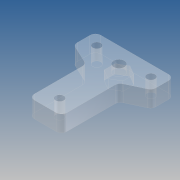
# Autodesk Inventor part: adapterplatte
Saved by Autodesk Inventor 2011 (Build 150239000, 239)
## iProperties
Created: 2014-03-14
Part Number: adapterplatte
Document SubType Name: Modeling
Designer: Kretschmer
Density: 1 g/cm^3
Author: Kretschmer
Autodesk Inventor part; units mm, degrees
ref_plane "YZ Plane" through (0, 0, 0) normal (1, 0, 0) x (0, 1, 0)
ref_plane "XZ Plane" through (0, 0, 0) normal (0, 1, 0) x (-1, 0, 0)
ref_plane "XY Plane" through (0, 0, 0) normal (0, 0, 1) x (1, 0, 0)
sketch "Skizze1" plane through (0, 0, 0) normal (0, 0, 1) x (1, 0, 0)
  line L0 (-14.5, -16.5) -> (14.5, -16.5)
  line L1 (14.5, -16.5) -> (14.5, 16.5)
  line L2 (14.5, 16.5) -> (-14.5, 16.5)
  line L3 (-14.5, 16.5) -> (-14.5, -16.5)
  point P0 (0, 0)
  point P1 (-14.5, 0)
  point P2 (0, -16.5)
  dimension "d0" = 29
  dimension "d1" = 33
  constraints: 8 end point, 2 midpoint, 2 parallel, 1 horizontal, 1 horizontal alignment, 1 perpendicular, 1 vertical alignment
  measures "d0" distance between parallel lines of L1 L3
  measures "d1" distance between parallel lines of L0 L2
extrude "Extrusion1" add sketch "Skizze1" along normal blind 6
hole "Hole1" at (-10, 12.5, 6) direction (0, 0, -1) diameter 3 end through all
pattern_linear "Rechteckige Anordnung1" count 2 spacing 20 along (1, 0, 0) of "Hole1"
sketch "Skizze2" plane through (0, 0, 6) normal (0, 0, 1) x (1, 0, 0)
  circle A0 centre (-10, 12.5) radius 3 projected
  line L0 (14.5, -16.5) -> (-14.5, -16.5) projected
  line L1 (-14.5, 16.5) -> (14.5, 16.5) projected
  line L2 (0, 16.5) -> (0, -16.5)
  circle A1 centre (10, 12.5) radius 1.5 projected
  point P0 (0, 0)
  point P1 (0, -11.2)
  dimension "d42" = 23.7
  constraints: 2 end point, 2 midpoint, 1 point on line
  measures "d42" vertical distance of A1.centre point (0, -11.2)
hole "Hole2" at (0, -11.2, 6) at (-10, 12.5, 6) direction (0, 0, -1) diameter 3 end through all
sketch "Skizze3" plane through (0, 0, 0) normal (0, 0, -1) x (-1, 0, 0)
  line L0 (14.5, -16.5) -> (-14.5, -16.5) projected
  line L1 (-14.5, 16.5) -> (14.5, 16.5) projected
  line L2 (0, -16.5) -> (0, 16.5)
  point P0 (0, 0)
  point P1 (0, 10.7)
  dimension "d24" = 5.8
  constraints: 2 end point, 2 midpoint, 1 point on line
  measures "d24" distance from line of L1 point (0, 10.7)
hole "Hole3" at (0, 10.7, 0) direction (0, 0, 1) diameter 4 end through all
sketch "Skizze4" plane through (0, 0, 0) normal (0, 0, -1) x (-1, 0, 0)
  circle A0 centre (0, 10.7) radius 2 projected
  line L0 (0, 6.6585) -> (-3.5, 8.6793)
  line L1 (-3.5, 8.6793) -> (-3.5, 12.7207)
  line L2 (-3.5, 12.7207) -> (0, 14.7415)
  line L3 (0, 14.7415) -> (3.5, 12.7207)
  line L4 (3.5, 12.7207) -> (3.5, 8.6793)
  line L5 (3.5, 8.6793) -> (0, 6.6585)
  point P0 (0, 0)
  dimension "d32" = 7
  constraints: 12 end point, 1 coincident, 13 other
  measures "d32" distance between parallel lines of L2 L5
extrude "Extrusion2" cut sketch "Skizze4" against normal blind 3.3
sketch "Skizze5" plane through (0, 0, 6) normal (0, 0, 1) x (1, 0, 0)
  line L0 (-14.5, -16.5) -> (-14.5, 16.5) projected
  line L1 (14.5, -16.5) -> (-14.5, -16.5) projected
  line L2 (-14.5, 16.5) -> (14.5, 16.5) projected
  line L3 (-14.5, 8.5) -> (-6, 4.5)
  line L4 (-6, 4.5) -> (-6, -16.5)
  line L5 (0, 16.5) -> (0, -16.5)
  line L6 (14.5, -16.5) -> (14.5, 16.5)
  line L7 (-14.5, -16.5) -> (14.5, -16.5)
  line L8 (14.5, 8.5) -> (6, 4.5)
  line L9 (6, 4.5) -> (6, -16.5)
  point P0 (0, 0)
  dimension "d36" = 12
  dimension "d37" = 8
  dimension "d38" = 6
  constraints: 14 end point, 5 symmetric about line, 4 point on line, 2 midpoint, 1 perpendicular
  measures "d36" distance from line of L2 L3.end
  measures "d37" distance of L0.end L3.start
  measures "d38" distance between parallel lines of L4 L5
extrude "Extrusion3" cut sketch "Skizze5" against normal blind 6 contours L0 L3 L4 L1 | L9 L8 L6 L1
fillet "Rundung1" radius 2 8 edges at (6, 4.5, 3) (6, -16.5, 3) (-6, -16.5, 3) (-6, 4.5, 3) (-14.5, 8.5, 3) (-14.5, 16.5, 3) (14.5, 16.5, 3) (14.5, 8.5, 3)
